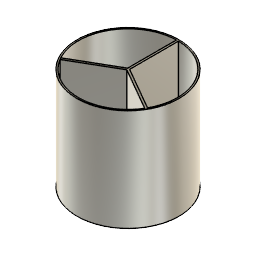
Trash bin IMP (Autodesk Fusion 360 design; units mm, degrees)
part number: 2026-03-01-21-54-43-821
Autodesk Fusion 360 part; units mm, degrees
sketch "Sketch1" plane through (0, 0, 0) normal (0, 0, 1) x (1, 0, 0)
  circle A0 centre (0, 0) radius 100
  dimension "d1" = 200
  constraint coincident A0.centre origin
  measures "d1" diameter of A0
extrude "Extrude1" add sketch "Sketch1" along normal blind 3
sketch "Sketch2" plane through (0, 0, 3) normal (0, 0, 1) x (-1, 0, 0)
  circle A0 centre (0, 0) radius 100
  circle A1 centre (0, 0) radius 100 construction
  circle A2 centre (0, 0) radius 100
  circle A3 centre (0, 0) radius 97
  dimension "d4" = 194
  constraint coincident A0.centre A1.centre
  constraint concentric A1 A2
  constraint concentric A2 A3
  measures "d4" diameter of A3
extrude "Extrude2" add sketch "Sketch2" along normal blind 220
sketch "Sketch3" plane through (0, 0, 3) normal (0, 0, 1) x (-1, 0, 0)
  circle A0 centre (0, 0) radius 97
  circle A1 centre (0, 0) radius 97 construction
  circle A2 centre (0, 0) radius 50 construction
  line L0 (0, 0) -> (0, -50) construction
  line L1 (0, 0) -> (-43.3013, 25) construction
  line L2 (0, 0) -> (43.3013, 25) construction
  line L3 (0, 0) -> (50, 0) construction
  circle A3 centre (0, 0) radius 2
  line L4 (-2, 0) -> (-2, -49.96)
  line L5 (2, 0) -> (2, -49.96)
  line L6 (0, 0) -> (-1, -1.7321) construction
  line L7 (0, 0) -> (1, 1.7321) construction
  line L8 (-1, -1.7321) -> (-44.2666, 23.2479)
  line L9 (1, 1.7321) -> (-42.2666, 26.712)
  line L10 (25.5472, 14.7497) -> (24.5472, 16.4818) construction
  line L11 (24.5472, 16.4818) -> (26.5472, 13.0177) construction
  line L12 (24.5472, 16.4818) -> (-70.6745, -38.4945) construction
  line L13 (-70.6745, -38.4945) -> (68.8541, 42.0623) construction
  line L14 (26.5472, 13.0177) -> (-23.3711, -15.8027) construction
  line L15 (-23.3711, -15.8027) -> (75.9084, 41.5164) construction
  line L16 (42.2666, 26.712) -> (-0.9955, 1.7346)
  line L17 (44.263, 23.2458) -> (2, -1.1547)
  arc A4 (44.263, 23.2458) -> (42.2666, 26.712) centre (2.1369, 1.2914) ccw
  line L18 (2, -49.96) -> (2, -96.9794)
  line L19 (-2, -49.96) -> (-2, -96.9794)
  line L20 (-44.2666, 23.2479) -> (-84.9866, 46.7576)
  line L21 (-42.2666, 26.712) -> (-82.9866, 50.2217)
  line L22 (42.2666, 26.712) -> (82.9856, 50.2212)
  line L23 (44.263, 23.2458) -> (84.9866, 46.7576)
  arc A5 (84.9866, 46.7576) -> (82.9856, 50.2212) centre (0.3022, 0.1428) ccw
  arc A6 (-2, -96.9794) -> (2, -96.9794) centre (0, -0.3234) ccw
  arc A7 (-82.9866, 50.2217) -> (-84.9866, 46.7576) centre (-0.2887, 0.1667) ccw
  dimension "d7" = 100
  dimension "d8" = 60
  dimension "d9" = 50
  dimension "d10" = 30
  dimension "d11" = 50
  dimension "d12" = 4
  dimension "d13" = 2
  dimension "d14" = 4
  dimension "d19" = 194
  constraint coincident A0.centre A1.centre
  constraint concentric A1 A2
  constraint coincident A2 L0.end
  constraint vertical L0
  constraint horizontal L3
  constraint coincident A3 L4.start
  constraint coincident A2 L4.end
  constraint parallel L0 L4
  constraint coincident A3 L5.start
  constraint coincident L3 L5.start
  constraint coincident A2 L5.end
  constraint perpendicular L3 L5
  constraint coincident A3 L6.end
  constraint perpendicular L1 L6
  constraint coincident A3 L7.end
  constraint parallel L6 L7
  constraint coincident A2 L8.end
  constraint tangent A3 L8
  constraint coincident A2 L9.end
  constraint tangent A3 L9
  constraint coincident L2 L10.start
  constraint perpendicular L2 L10
  constraint perpendicular L2 L11
  constraint perpendicular L10 L12
  constraint perpendicular L11 L13
  constraint perpendicular L11 L14
  constraint perpendicular L11 L15
  constraint coincident A2 L16.start
  constraint coincident L13 L16.start
  constraint coincident L12 L16.end
  constraint coincident L15 L17.start
  constraint coincident L5 L17.end
  constraint coincident L15 L17.end
  constraint coincident L2.end A4
  constraint coincident A1 L18.end
  constraint parallel L5 L18
  constraint coincident A1 L19.end
  constraint parallel L18 L19
  constraint coincident A1 L20.end
  constraint parallel L8 L20
  constraint coincident A1 L21.end
  constraint parallel L9 L21
  constraint parallel L13 L22
  constraint coincident A0 L23.end
  constraint parallel L15 L23
  measures "d7" diameter of A2
  measures "d8" angle of L0 L1
  measures "d9" distance of A0.centre L1.end
  measures "d10" angle of L2 L3
  measures "d11" distance of A0.centre L2.end
  measures "d12" diameter of A3
  measures "d13" distance of L10.start L10.end
  measures "d14" distance of L10.end L11.end
  measures "d19" diameter of A1
extrude "Extrude3" add sketch "Sketch3" along normal blind 220 contours A4 L22 L23 A5 | A0 A3 L4 L5 L8 L18 L19 A6 | A0 A3 L4 L8 L9 L16 L20 L21 A7 | A3 L5 L9 L16 L17 A4 | A3 L9 L16 | A3 | A3 L4 L8
extrude "Extrude5" cut 1 faces at (0, 0, 223) along direction (0, 0, -1) blind 23
sketch "Sketch4" plane through (0, 0, 0) normal (0, 0, -1) x (1, 0, 0)
  circle A0 centre (0, 0) radius 100
  circle A1 centre (0, 0) radius 2 construction
  line L0 (24.5472, 16.4818) -> (-70.6745, -38.4945) construction
  line L1 (-23.3711, -15.8027) -> (75.9084, 41.5164) construction
  line L2 (-1, 1.7321) -> (-5.3301, -0.7679) construction
  line L3 (-1, 1.7321) -> (1, -1.7321) construction
  line L4 (1, -1.7321) -> (-3.3301, -4.2321) construction
  line L5 (-3.3301, -4.2321) -> (-5.3301, -0.7679) construction
  line L6 (-4.3301, -2.5) -> (0, 0) construction
  line L7 (0, 0) -> (1.5155, 0.875) construction
  line L8 (1.5155, 0.875) -> (0.5155, 2.6071) construction
  line L9 (1.5155, 0.875) -> (2.5155, -0.8571) construction
  line L10 (1.5155, 0.875) -> (0.7655, 2.174) construction
  line L11 (1.5155, 0.875) -> (2.2655, -0.424) construction
  line L12 (0.7655, 2.174) -> (2.2655, -0.424) construction
  line L13 (2.2655, -0.424) -> (-0.7655, -2.174) construction
  line L14 (0.7655, 2.174) -> (-2.2655, 0.424) construction
  line L15 (-2.2655, 0.424) -> (-0.7655, -2.174) construction
  line L16 (0, 0) -> (4.3301, 2.5) construction
  line L17 (1.5155, 0.875) -> (2.2084, 1.275) construction
  arc A2 (2.2655, -0.424) -> (0.7655, 2.174) centre (0.6441, 0.3719) ccw construction
  line L18 (-1.5155, -0.875) -> (-2.2084, -1.275) construction
  arc A3 (-2.2655, 0.424) -> (-0.7655, -2.174) centre (-0.6441, -0.3719) ccw construction
  line L19 (0, 0) -> (-0.8, 1.3856) construction
  line L20 (0, 0) -> (0.8, -1.3856) construction
  line L21 (-0.8, 1.3856) -> (0.7155, 2.2606)
  line L22 (-0.8, 1.3856) -> (-2.3155, 0.5106)
  line L23 (-2.3155, 0.5106) -> (-0.7155, -2.2606) construction
  line L24 (-0.7155, -2.2606) -> (2.3155, -0.5106)
  line L25 (0, 0) -> (2.2517, 1.3) construction
  line L26 (0, 0) -> (-2.2517, -1.3) construction
  arc A4 (2.3155, -0.5106) -> (0.7155, 2.2606) centre (0.5795, 0.3346) ccw
  arc A5 (-2.3155, 0.5106) -> (-0.7155, -2.2606) centre (-0.5795, -0.3346) ccw
  dimension "d22" = 4
  dimension "d23" = 5
  dimension "d24" = 4
  dimension "d25" = 5
  dimension "d26" = 1.75
  dimension "d27" = 1.5
  dimension "d28" = 1.5
  dimension "d29" = 3.5
  dimension "d30" = 3.5
  dimension "d31" = 5
  dimension "d32" = 0.8
  dimension "d33" = 0.8
  dimension "d34" = 1.6
  dimension "d35" = 1.6
  dimension "d36" = 1.75
  dimension "d37" = 1.75
  dimension "d38" = 3.2
  dimension "d39" = 3.5
  dimension "d40" = 2.6
  dimension "d41" = 2.6
  constraint coincident A0.centre A1.centre
  constraint coincident L0 L2.start
  constraint coincident A1 L2.start
  constraint parallel L0 L2
  constraint coincident L1 L3.end
  constraint coincident A1 L3.end
  constraint perpendicular L3 L4
  constraint perpendicular L2 L5
  constraint midpoint L5 L6.start
  constraint perpendicular L3 L7
  constraint coincident L0 L8.end
  constraint perpendicular L0 L8
  constraint coincident L1 L9.end
  constraint perpendicular L1 L9
  constraint perpendicular L7 L10
  constraint perpendicular L7 L11
  constraint perpendicular L11 L13
  constraint perpendicular L3 L14
  constraint perpendicular L3 L16
  constraint perpendicular L12 L17
  constraint coincident L17.end A2
  constraint midpoint L15 L18.start
  constraint perpendicular L15 L18
  constraint coincident L18.end A3
  constraint perpendicular L7 L19
  constraint perpendicular L1 L20
  constraint perpendicular L19 L21
  constraint perpendicular L19 L22
  constraint perpendicular L6 L23
  constraint perpendicular L3 L24
  constraint parallel L16 L25
  constraint perpendicular L3 L26
  constraint coincident L25.end A4
  constraint coincident L26.end A5
  measures "d22" diameter of A1
  measures "d23" distance of L2.start L2.end
  measures "d24" distance of L2.start L3.end
  measures "d25" distance of L3.end L4.end
  measures "d26" distance of A0.centre L7.end
  measures "d27" distance of L7.end L10.end
  measures "d28" distance of L7.end L11.end
  measures "d29" distance of L11.end L13.end
  measures "d30" distance of L10.end L14.end
  measures "d31" distance of A0.centre L16.end
  measures "d32" distance of L7.end L17.end
  measures "d33" distance of L18.start L18.end
  measures "d34" distance of A0.centre L19.end
  measures "d35" distance of A0.centre L20.end
  measures "d36" distance of L19.end L21.end
  measures "d37" distance of L19.end L22.end
  measures "d38" distance of L22.end L23.end
  measures "d39" distance of L23.end L24.end
  measures "d40" distance of A0.centre L25.end
  measures "d41" distance of A0.centre L26.end
extrude "Extrude6" cut sketch "Sketch4" against normal blind 6 contours L21 L22 L24 A4 A5
